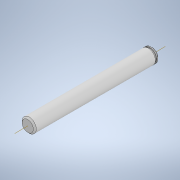
# Autodesk Inventor part: Shaft
Saved by Autodesk Inventor 2021 (Build 250183000, 183)
## iProperties
Created: 2022-01-12
Part Number: Shaft
Material: Generic
Document SubType Name: Modeling
Designer: stefi
Density: 1 g/cm^3
Appearance: Default
Author: stefi
Autodesk Inventor part; units mm, degrees
ref_plane "YZ Plane" through (0, 0, 0) normal (1, 0, 0) x (0, 1, 0)
ref_plane "XZ Plane" through (0, 0, 0) normal (0, 1, 0) x (-1, 0, 0)
ref_plane "XY Plane" through (0, 0, 0) normal (0, 0, 1) x (1, 0, 0)
sketch "Sketch1" plane through (0, 0, 0) normal (0, 0, 1) x (1, 0, 0)
  circle A0 centre (0, 0) radius 4.825
  dimension "d0" = 9.65
  constraints: 1 centre point, 1 coincident
  measures "d0" diameter of A0
extrude "Extrusion1" add sketch "Sketch1" along normal blind 85
chamfer "Chamfer1" distance 1 angle 45 2 edges at (-4.825, 0, 85) (-4.825, 0, 0)
sketch "Sketch2" plane through (0, 0, 0) normal (0, 1, 0) x (-1, 0, 0)
  line L0 (4.825, 1) -> (4.825, 84) projected
  line L1 (4.825, 1.69) -> (4.325, 1.69)
  line L2 (4.325, 1.69) -> (4.325, 2.67)
  line L3 (4.325, 2.67) -> (4.825, 2.67)
  line L4 (4.825, 2.67) -> (4.825, 1.69)
  line L5 (0, -17) -> (0, 102) projected
  point P0 (0, 0)
  dimension "d6" = 0.5
  dimension "d7" = 0.98
  dimension "d8" = 0.69
  constraints: 8 end point, 2 parallel, 1 horizontal, 1 perpendicular, 1 point on line
  measures "d6" distance of L2.end L3.end
  measures "d7" distance of L1.end L2.end
  measures "d8" distance of L0.start L1.start
revolve "Revolution1" cut sketch "Sketch2" angle 360 about axis through (0, 0, -10) along (0, 0, 1)
body "Solid1"
